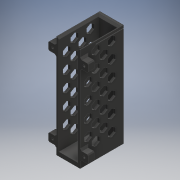
# Autodesk Inventor part: LiFeGuard
Saved by Autodesk Inventor 2018.3 (Build 223284000, 284)
## iProperties
Created: 2018-08-27
Part Number: LiFeGuard
Material: ABS プラスチック
Document SubType Name: Modeling
Designer: shun2
Density: 1.06 g/cm^3
Appearance: 滑らか - 黒
Author: shun2
Autodesk Inventor part; units mm, degrees
ref_plane "YZ Plane" through (0, 0, 0) normal (1, 0, 0) x (0, 1, 0)
ref_plane "XZ Plane" through (0, 0, 0) normal (0, 1, 0) x (-1, 0, 0)
ref_plane "XY Plane" through (0, 0, 0) normal (0, 0, 1) x (1, 0, 0)
sketch "スケッチ1" plane through (0, 0, 0) normal (0, 0, 1) x (1, 0, 0)
  line L0 (30, 0) -> (30, 55)
  line L1 (30, 55) -> (0, 55)
  line L2 (0, 55) -> (0, 2)
  line L3 (0, 2) -> (0, 0)
  line L4 (0, 2) -> (0, 0)
  line L5 (0, 0) -> (2, 0)
  line L6 (30, 2) -> (30, 0)
  line L7 (30, 0) -> (28, 0)
  line L8 (0, 55) -> (3, 55)
  line L9 (3, 0) -> (0, 0)
  line L10 (0, 0) -> (0, 55)
  line L11 (30, 55) -> (27, 55)
  line L12 (27, 50) -> (27, 0)
  line L13 (27, 0) -> (30, 0)
  line L14 (30, 0) -> (30, 55)
  line L15 (0, 55) -> (30, 55)
  line L16 (30, 55) -> (30, 50)
  line L17 (27, 50) -> (3, 50)
  line L18 (0, 50) -> (0, 55)
  line L19 (3, 50) -> (3, 0)
  dimension "d57" = 3
  dimension "d58" = 3
  dimension "d59" = 5
  constraints: 40 end point, 7 parallel, 3 horizontal, 3 perpendicular, 2 point on line, 1 vertical
  measures "d57" distance of L9.start L9.end
  measures "d58" distance of L13.end L12.end
  measures "d59" distance of L15.end L16.end
extrude "押し出し1" add sketch "スケッチ1" along normal blind 130
sketch "スケッチ4" plane through (0, 0, 0) normal (0, 0, -1) x (-1, 0, 0)
  line L0 (-30, 0) -> (-30, 55) projected
  line L1 (-30, 55) -> (0, 55)
  line L2 (0, 55) -> (0, 0)
  line L3 (0, 0) -> (-30, 0)
  line L4 (-30, 0) -> (-30, 55)
  constraints: 8 end point, 2 parallel, 1 horizontal, 1 perpendicular
extrude "押し出し5" add sketch "スケッチ4" against normal blind 5
sketch "スケッチ5" plane through (30, 0, 130) normal (1, 0, 0) x (0, 0, -1)
  line L0 (130, 55) -> (0, 55) projected
  line L1 (0, 0) -> (0, 55) projected
  line L2 (130, 0) -> (0, 0) projected
  line L3 (130, 55) -> (130, 0) projected
  line L4 (0, 0) -> (0, 55) projected
  line L5 (22.8868, 15) -> (25.7735, 10)
  line L6 (25.7735, 10) -> (22.8868, 5)
  line L7 (22.8868, 5) -> (17.1132, 5)
  line L8 (17.1132, 5) -> (14.2265, 10)
  line L9 (14.2265, 10) -> (17.1132, 15)
  line L10 (17.1132, 15) -> (22.8868, 15)
  line L11 (42.8868, 15) -> (45.7735, 10)
  line L12 (45.7735, 10) -> (42.8868, 5)
  line L13 (42.8868, 5) -> (37.1132, 5)
  line L14 (37.1132, 5) -> (34.2265, 10)
  line L15 (34.2265, 10) -> (37.1132, 15)
  line L16 (37.1132, 15) -> (42.8868, 15)
  line L17 (62.8868, 15) -> (65.7735, 10)
  line L18 (65.7735, 10) -> (62.8868, 5)
  line L19 (62.8868, 5) -> (57.1132, 5)
  line L20 (57.1132, 5) -> (54.2265, 10)
  line L21 (54.2265, 10) -> (57.1132, 15)
  line L22 (57.1132, 15) -> (62.8868, 15)
  line L23 (82.8868, 15) -> (85.7735, 10)
  line L24 (85.7735, 10) -> (82.8868, 5)
  line L25 (82.8868, 5) -> (77.1132, 5)
  line L26 (77.1132, 5) -> (74.2265, 10)
  line L27 (74.2265, 10) -> (77.1132, 15)
  line L28 (77.1132, 15) -> (82.8868, 15)
  line L29 (102.8868, 15) -> (105.7735, 10)
  line L30 (105.7735, 10) -> (102.8868, 5)
  line L31 (102.8868, 5) -> (97.1132, 5)
  line L32 (97.1132, 5) -> (94.2265, 10)
  line L33 (94.2265, 10) -> (97.1132, 15)
  line L34 (97.1132, 15) -> (102.8868, 15)
  line L35 (12.8868, 25) -> (15.7735, 20)
  line L36 (15.7735, 20) -> (12.8868, 15)
  line L37 (12.8868, 15) -> (7.1132, 15)
  line L38 (7.1132, 15) -> (4.2265, 20)
  line L39 (4.2265, 20) -> (7.1132, 25)
  line L40 (7.1132, 25) -> (12.8868, 25)
  line L41 (32.8868, 25) -> (35.7735, 20)
  line L42 (35.7735, 20) -> (32.8868, 15)
  line L43 (32.8868, 15) -> (27.1132, 15)
  line L44 (27.1132, 15) -> (24.2265, 20)
  line L45 (24.2265, 20) -> (27.1132, 25)
  line L46 (27.1132, 25) -> (32.8868, 25)
  line L47 (52.8868, 25) -> (55.7735, 20)
  line L48 (55.7735, 20) -> (52.8868, 15)
  line L49 (52.8868, 15) -> (47.1132, 15)
  line L50 (47.1132, 15) -> (44.2265, 20)
  line L51 (44.2265, 20) -> (47.1132, 25)
  line L52 (47.1132, 25) -> (52.8868, 25)
  line L53 (72.8868, 25) -> (75.7735, 20)
  line L54 (75.7735, 20) -> (72.8868, 15)
  line L55 (72.8868, 15) -> (67.1132, 15)
  line L56 (67.1132, 15) -> (64.2265, 20)
  line L57 (64.2265, 20) -> (67.1132, 25)
  line L58 (67.1132, 25) -> (72.8868, 25)
  line L59 (92.8868, 25) -> (95.7735, 20)
  line L60 (95.7735, 20) -> (92.8868, 15)
  line L61 (92.8868, 15) -> (87.1132, 15)
  line L62 (87.1132, 15) -> (84.2265, 20)
  line L63 (84.2265, 20) -> (87.1132, 25)
  line L64 (87.1132, 25) -> (92.8868, 25)
  line L65 (112.8868, 25) -> (115.7735, 20)
  line L66 (115.7735, 20) -> (112.8868, 15)
  line L67 (112.8868, 15) -> (107.1132, 15)
  line L68 (107.1132, 15) -> (104.2265, 20)
  line L69 (104.2265, 20) -> (107.1132, 25)
  line L70 (107.1132, 25) -> (112.8868, 25)
  line L71 (22.8868, 35) -> (25.7735, 30)
  line L72 (25.7735, 30) -> (22.8868, 25)
  line L73 (22.8868, 25) -> (17.1132, 25)
  line L74 (17.1132, 25) -> (14.2265, 30)
  line L75 (14.2265, 30) -> (17.1132, 35)
  line L76 (17.1132, 35) -> (22.8868, 35)
  line L77 (42.8868, 35) -> (45.7735, 30)
  line L78 (45.7735, 30) -> (42.8868, 25)
  line L79 (42.8868, 25) -> (37.1132, 25)
  line L80 (37.1132, 25) -> (34.2265, 30)
  line L81 (34.2265, 30) -> (37.1132, 35)
  line L82 (37.1132, 35) -> (42.8868, 35)
  line L83 (62.8868, 35) -> (65.7735, 30)
  line L84 (65.7735, 30) -> (62.8868, 25)
  line L85 (62.8868, 25) -> (57.1132, 25)
  line L86 (57.1132, 25) -> (54.2265, 30)
  line L87 (54.2265, 30) -> (57.1132, 35)
  line L88 (57.1132, 35) -> (62.8868, 35)
  line L89 (82.8868, 35) -> (85.7735, 30)
  line L90 (85.7735, 30) -> (82.8868, 25)
  line L91 (82.8868, 25) -> (77.1132, 25)
  line L92 (77.1132, 25) -> (74.2265, 30)
  line L93 (74.2265, 30) -> (77.1132, 35)
  line L94 (77.1132, 35) -> (82.8868, 35)
  line L95 (102.8868, 35) -> (105.7735, 30)
  line L96 (105.7735, 30) -> (102.8868, 25)
  line L97 (102.8868, 25) -> (97.1132, 25)
  line L98 (97.1132, 25) -> (94.2265, 30)
  line L99 (94.2265, 30) -> (97.1132, 35)
  line L100 (97.1132, 35) -> (102.8868, 35)
  line L101 (0, 55) -> (0, 0) projected
  line L102 (12.8868, 45) -> (15.7735, 40)
  line L103 (15.7735, 40) -> (12.8868, 35)
  line L104 (12.8868, 35) -> (7.1132, 35)
  line L105 (7.1132, 35) -> (4.2265, 40)
  line L106 (4.2265, 40) -> (7.1132, 45)
  line L107 (7.1132, 45) -> (12.8868, 45)
  line L108 (32.8868, 45) -> (35.7735, 40)
  line L109 (35.7735, 40) -> (32.8868, 35)
  line L110 (32.8868, 35) -> (27.1132, 35)
  line L111 (27.1132, 35) -> (24.2265, 40)
  line L112 (24.2265, 40) -> (27.1132, 45)
  line L113 (27.1132, 45) -> (32.8868, 45)
  line L114 (52.8868, 45) -> (55.7735, 40)
  line L115 (55.7735, 40) -> (52.8868, 35)
  line L116 (52.8868, 35) -> (47.1132, 35)
  line L117 (47.1132, 35) -> (44.2265, 40)
  line L118 (44.2265, 40) -> (47.1132, 45)
  line L119 (47.1132, 45) -> (52.8868, 45)
  line L120 (72.8868, 45) -> (75.7735, 40)
  line L121 (75.7735, 40) -> (72.8868, 35)
  line L122 (72.8868, 35) -> (67.1132, 35)
  line L123 (67.1132, 35) -> (64.2265, 40)
  line L124 (64.2265, 40) -> (67.1132, 45)
  line L125 (67.1132, 45) -> (72.8868, 45)
  line L126 (92.8868, 45) -> (95.7735, 40)
  line L127 (95.7735, 40) -> (92.8868, 35)
  line L128 (92.8868, 35) -> (87.1132, 35)
  line L129 (87.1132, 35) -> (84.2265, 40)
  line L130 (84.2265, 40) -> (87.1132, 45)
  line L131 (87.1132, 45) -> (92.8868, 45)
  line L132 (112.8868, 45) -> (115.7735, 40)
  line L133 (115.7735, 40) -> (112.8868, 35)
  line L134 (112.8868, 35) -> (107.1132, 35)
  line L135 (107.1132, 35) -> (104.2265, 40)
  line L136 (104.2265, 40) -> (107.1132, 45)
  line L137 (107.1132, 45) -> (112.8868, 45)
  point P0 (20, 10)
  point P1 (20, 15)
  point P2 (40, 10)
  point P3 (40, 15)
  point P4 (60, 10)
  point P5 (60, 15)
  point P6 (80, 10)
  point P7 (80, 15)
  point P8 (100, 10)
  point P9 (100, 15)
  point P10 (0, 50)
  point P11 (125, 50)
  point P12 (10, 25)
  point P13 (30, 25)
  point P14 (50, 25)
  point P15 (70, 25)
  point P16 (90, 25)
  point P17 (110, 25)
  point P18 (20, 30)
  point P19 (20, 35)
  point P20 (40, 30)
  point P21 (40, 35)
  point P22 (60, 30)
  point P23 (60, 35)
  point P24 (80, 30)
  point P25 (80, 35)
  point P26 (100, 30)
  point P27 (100, 35)
  point P28 (10, 40)
  point P29 (10, 45)
  point P30 (30, 40)
  point P31 (30, 45)
  point P32 (50, 40)
  point P33 (50, 45)
  point P34 (70, 40)
  point P35 (70, 45)
  point P36 (90, 40)
  point P37 (90, 45)
  point P38 (110, 40)
  point P39 (110, 45)
  constraints: 264 end point, 22 midpoint, 1 point on line, 208 other
extrude "押し出し6" cut sketch "スケッチ5" against normal blind 50 contours L5 L6 L7 L8 L9 L10 | L11 L12 L13 L14 L15 L16 | L17 L18 L19 L20 L21 L22 | L23 L24 L25 L26 L27 L28 | L29 L30 L31 L32 L33 L34 | L35 L36 L37 L38 L39 L40 | L41 L42 L43 L44 L45 L46 | L47 L48 L49 L50 L51 L52 | L53 L54 L55 L56 L57 L58 | L59 L60 L61 L62 L63 L64 | L65 L66 L67 L68 L69 L70 | L71 L72 L73 L74 L75 L76 | L77 L78 L79 L80 L81 L82 | L83 L84 L85 L86 L87 L88 | L89 L90 L91 L92 L93 L94 | L95 L96 L97 L98 L99 L100 | L102 L103 L104 L105 L106 L107 | L108 L109 L110 L111 L112 L113 | L114 L115 L116 L117 L118 L119 | L120 L121 L122 L123 L124 L125 | L126 L127 L128 L129 L130 L131 | L132 L133 L134 L135 L136 L137
chamfer "面取り4" distance 2 angle 45 3 edges at (15, 50, 130) (3, 25, 130) (27, 25, 130)
sketch "スケッチ6" plane through (0, 0, 0) normal (0, -1, 0) x (1, 0, 0)
  line L0 (0, 0) -> (0, 130) projected
  line L1 (0, 10) -> (-10, 10)
  line L2 (-10, 10) -> (-10, 20)
  line L3 (-10, 20) -> (0, 20)
  line L4 (0, 20) -> (0, 10)
  line L5 (0, 120) -> (-10, 120)
  line L6 (-10, 120) -> (-10, 110)
  line L7 (-10, 110) -> (0, 110)
  line L8 (0, 110) -> (0, 120)
  line L9 (30, 120) -> (40, 120)
  line L10 (40, 120) -> (40, 110)
  line L11 (40, 110) -> (30, 110)
  line L12 (30, 110) -> (30, 120)
  line L13 (30, 0) -> (30, 130) projected
  line L14 (30, 20) -> (40, 20)
  line L15 (40, 20) -> (40, 10)
  line L16 (40, 10) -> (30, 10)
  line L17 (30, 10) -> (30, 20)
  circle A0 centre (-5, 15) radius 1.5
  circle A1 centre (35, 15) radius 1.5
  circle A2 centre (35, 115) radius 1.5
  circle A3 centre (-5, 115) radius 1.5
  dimension "d71" = 10
  dimension "d72" = 10
  dimension "d73" = 10
  dimension "d74" = 10
  dimension "d75" = 10
  dimension "d76" = 10
  dimension "d77" = 10
  dimension "d78" = 10
  dimension "d90" = 3
  dimension "d91" = 3
  dimension "d92" = 3
  dimension "d93" = 3
  constraints: 32 end point, 8 parallel, 4 centre point, 4 horizontal, 4 perpendicular, 3 point on line
  measures "d71" distance of L2.end L3.end
  measures "d72" distance of L1.end L2.end
  measures "d73" distance of L7.end L6.end
  measures "d74" distance of L6.end L5.end
  measures "d75" distance of L10.end L11.end
  measures "d76" distance of L9.end L10.end
  measures "d77" distance of L15.end L16.end
  measures "d78" distance of L14.end L15.end
  measures "d90" diameter of A0
  measures "d91" diameter of A1
  measures "d92" diameter of A2
  measures "d93" diameter of A3
extrude "押し出し7" add sketch "スケッチ6" against normal blind 8
chamfer "面取り5" distance 2 angle 45 8 edges at (0, 4, 120) (0, 4, 20) (0, 2.5, 110) (0, 4, 10) (30, 2.5, 110) (30, 4, 10) (30, 4, 20) (30, 4, 120)
chamfer "面取り6" distance 2 angle 45 10 edges at (30, 8, 121) (30, 8, 117.3094) (30, 8, 9) (30, 8, 15) (30, 8, 21) (0, 8, 9) (0, 8, 15) (0, 8, 21) (0, 8, 121) (0, 8, 117.3094)
chamfer "面取り7" distance 1 angle 45 8 edges at (-10, 4, 10) (-10, 4, 20) (-10, 4, 110) (-10, 4, 120) (40, 4, 120) (40, 4, 110) (40, 4, 20) (40, 4, 10)
sketch "スケッチ7" plane through (0, 55, 130) normal (0, 1, 0) x (1, 0, 0)
  line L0 (0, 130) -> (0, 0) projected
  line L1 (30, 130) -> (30, 0) projected
  line L2 (0, 4) -> (1, 4)
  line L3 (30, 0) -> (0, 0) projected
  line L4 (1, 4) -> (0, 3)
  line L5 (30, 4) -> (29, 4)
  line L6 (29, 4) -> (30, 3)
  dimension "d96" = 1
  dimension "d97" = 45
  dimension "d99" = 1
  constraints: 8 end point, 4 point on line, 1 horizontal, 1 parallel
  measures "d96" distance of L2.start L2.end
  measures "d97" angle of L2 L4
  measures "d99" distance of L5.start L5.end
extrude "押し出し8" cut sketch "スケッチ7" against normal blind 35
